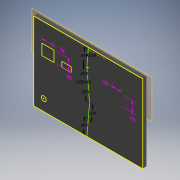
# Autodesk Inventor part: compnent box front
Saved by Autodesk Inventor 2021 (Build 250183000, 183)
## iProperties
Created: 2023-01-12
Part Number: compnent box front
Material: Generic
Document SubType Name: Modeling
Designer: boyle
Density: 1 g/cm^3
Appearance: Default
Author: boyle
Autodesk Inventor part; units mm, degrees
ref_plane "YZ Plane" through (0, 0, 0) normal (1, 0, 0) x (0, 1, 0)
ref_plane "XZ Plane" through (0, 0, 0) normal (0, 1, 0) x (-1, 0, 0)
ref_plane "XY Plane" through (0, 0, 0) normal (0, 0, 1) x (1, 0, 0)
ref_plane "Work Plane1" through (0, 0, 0) normal (0, 0, 1) x (1, 0, 0)
ref_plane "Work Plane2" through (-88.9, -98.425, 0) normal (0, 0, 1) x (1, 0, 0)
sketch "Sketch1" plane through (0, 0, 0) normal (0, 0, 1) x (1, 0, 0)
  line L0 (19.05, -98.425) -> (-88.9, -98.425) projected
  line L1 (-88.9, -98.425) -> (-88.9, -28.575) projected
  line L2 (-88.9, -28.575) -> (-88.9, 28.575) projected
  line L3 (-88.9, 28.575) -> (-85.09, 28.575) projected
  line L4 (88.9, 28.575) -> (88.9, -28.575) projected
  line L5 (85.09, 28.575) -> (88.9, 28.575) projected
  line L6 (19.05, -28.575) -> (19.05, -98.425) projected
  line L7 (-88.9, 28.575) -> (19.05, 28.575)
  line L8 (19.05, 28.575) -> (19.05, -98.425)
  line L9 (19.05, -98.425) -> (-88.9, -98.425)
  line L10 (-88.9, -98.425) -> (-88.9, 28.575)
  line L11 (15.24, -94.615) -> (-85.09, -94.615) projected
  line L12 (15.24, -94.615) -> (15.24, -28.575) projected
  line L13 (-85.09, -28.575) -> (15.24, -28.575) projected
  line L14 (-85.09, -94.615) -> (-85.09, -28.575) projected
  line L15 (19.05, -28.575) -> (19.05, -98.425) projected
  line L16 (15.24, -28.575) -> (19.05, -28.575) projected
  line L17 (-88.9, -98.425) -> (-88.9, -28.575) projected
  line L18 (19.05, -98.425) -> (-88.9, -98.425) projected
  line L19 (-88.9, 28.575) -> (88.9, 28.575) projected
  line L20 (-88.9, -28.575) -> (19.05, -28.575)
  line L21 (19.05, -28.575) -> (19.05, -98.425)
  line L22 (19.05, -98.425) -> (-88.9, -98.425)
  line L23 (-88.9, -98.425) -> (-88.9, -28.575)
  line L24 (88.9, 28.575) -> (88.9, -98.425)
  line L25 (88.9, -98.425) -> (19.05, -98.425)
  point P0 (0, 0)
  constraints: 20 end point, 4 parallel, 3 perpendicular, 2 horizontal, 1 vertical, 1 other
extrude "Extrusion1" add sketch "Sketch1" along normal blind 6.35 from surface at 0
sketch "Sketch2" plane through (0, 0, 6.35) normal (0, 0, 1) x (1, 0, 0)
  line L0 (-88.9, -98.425) -> (88.9, -98.425) projected
  line L1 (-88.9, -98.425) -> (-88.9, -28.575)
  line L2 (-88.9, 28.575) -> (-88.9, -98.425) projected
  line L3 (88.9, -98.425) -> (88.9, 28.575) projected
  circle A0 centre (-72.4784, -80.0377) radius 3.937
  line L4 (-88.9, 28.575) -> (88.9, 28.575)
  line L5 (88.9, 28.575) -> (88.9, -28.575)
  line L6 (-88.9, -28.575) -> (-88.9, 28.575)
  line L7 (88.9, 28.575) -> (-88.9, 28.575) projected
  line L8 (-43.0622, -12.632) -> (-27.8222, -12.632)
  line L9 (-27.8222, -12.632) -> (-27.8222, -20.76)
  line L10 (-27.8222, -20.76) -> (-43.0622, -20.76)
  line L11 (-43.0622, -20.76) -> (-43.0622, -12.632)
  line L12 (-43.0622, -12.632) -> (-27.8222, -20.76) construction
  line L13 (-27.8222, -12.632) -> (-43.0622, -20.76) construction
  line L14 (-75.5122, -3.16) -> (-55.7622, -3.16)
  line L15 (-55.7622, -3.16) -> (-55.7622, -20.76)
  line L16 (-55.7622, -20.76) -> (-75.5122, -20.76)
  line L17 (-75.5122, -20.76) -> (-75.5122, -3.16)
  line L18 (-75.5122, -3.16) -> (-55.7622, -20.76) construction
  line L19 (-55.7622, -3.16) -> (-75.5122, -20.76) construction
  line L20 (-62.5275, -46.3991) -> (-26.5275, -46.3991)
  line L21 (-26.5275, -46.3991) -> (-26.5275, -82.3991)
  line L22 (-26.5275, -82.3991) -> (-62.5275, -82.3991)
  line L23 (-62.5275, -46.3991) -> (-26.5275, -82.3991) construction
  line L24 (-26.5275, -46.3991) -> (-62.5275, -82.3991) construction
  line L25 (-62.5275, -46.3991) -> (-62.5275, -82.3991)
  line L26 (-44.5275, -46.3991) -> (-44.5275, -49.3991)
  line L27 (-44.5275, -49.3991) -> (-62.5275, -49.3991)
  line L28 (-44.5275, -49.3991) -> (-26.5275, -49.3991)
  line L29 (-44.5275, -49.3991) -> (-44.5275, -52.3991)
  line L30 (-44.5275, -52.3991) -> (-62.5275, -52.3991)
  line L31 (-44.5275, -52.3991) -> (-26.5275, -52.3991)
  line L32 (-44.5275, -52.3991) -> (-44.5275, -55.3991)
  line L33 (-44.5275, -55.3991) -> (-62.5275, -55.3991)
  line L34 (-44.5275, -55.3991) -> (-26.5275, -55.3991)
  line L35 (-44.5275, -55.3991) -> (-44.5275, -58.3991)
  line L36 (-44.5275, -58.3991) -> (-62.5275, -58.3991)
  line L37 (-44.5275, -58.3991) -> (-26.5275, -58.3991)
  line L38 (-44.5275, -58.3991) -> (-44.5275, -61.3991)
  line L39 (-44.5275, -61.3991) -> (-62.5275, -61.3991)
  line L40 (-44.5275, -61.3991) -> (-26.5275, -61.3991)
  line L41 (-44.5275, -61.3991) -> (-44.5275, -64.3991)
  line L42 (-44.5275, -64.3991) -> (-62.5275, -64.3991)
  line L43 (-44.5275, -64.3991) -> (-26.5275, -64.3991)
  line L44 (-44.5275, -64.3991) -> (-44.5275, -67.3991)
  line L45 (-44.5275, -67.3991) -> (-62.5275, -67.3991)
  line L46 (-44.5275, -67.3991) -> (-26.5275, -67.3991)
  line L47 (-44.5275, -67.3991) -> (-44.5275, -70.3991)
  line L48 (-44.5275, -70.3991) -> (-62.5275, -70.3991)
  line L49 (-44.5275, -70.3991) -> (-26.5275, -70.3991)
  line L50 (-44.5275, -70.3991) -> (-44.5275, -73.3991)
  line L51 (-44.5275, -73.3991) -> (-62.5275, -73.3991)
  line L52 (-44.5275, -73.3991) -> (-26.5275, -73.3991)
  line L53 (-44.5275, -73.3991) -> (-44.5275, -76.3991)
  line L54 (-44.5275, -76.3991) -> (-62.5275, -76.3991)
  line L55 (-44.5275, -76.3991) -> (-26.5275, -76.3991)
  line L56 (-44.5275, -76.3991) -> (-44.5275, -79.3991)
  line L57 (-44.5275, -79.3991) -> (-62.5275, -79.3991)
  line L58 (-44.5275, -79.3991) -> (-26.5275, -79.3991)
  line L59 (-44.5275, -79.3991) -> (-44.5275, -82.3991)
  line L60 (-44.5275, -82.3991) -> (-62.5275, -82.3991)
  line L61 (-44.5275, -82.3991) -> (-26.5275, -82.3991)
  line L62 (-43.0622, -20.76) -> (-55.7622, -20.76)
  point P0 (-65.6372, -11.96)
  point P1 (-62.5275, -67.3991)
  point P2 (-26.5275, -70.3991)
  point P3 (-26.5275, -67.3991)
  point P4 (-26.5275, -76.3991)
  point P5 (-26.5275, -73.3991)
  point P6 (-26.5275, -79.3991)
  point P7 (-26.5275, -61.3991)
  point P8 (-26.5275, -58.3991)
  point P9 (-26.5275, -55.3991)
  point P10 (-26.5275, -52.3991)
  dimension "d2" = 69.85
  dimension "d5" = 7.874
  dimension "d8" = 15.24
  dimension "d9" = 8.128
  dimension "d12" = 19.75
  dimension "d13" = 17.6
  dimension "d34" = 36
  dimension "d35" = 36
  dimension "d39" = 3
  dimension "d40" = 3
  dimension "d41" = 3
  dimension "d42" = 3
  dimension "d43" = 3
  dimension "d44" = 3
  dimension "d45" = 3
  dimension "d46" = 3
  dimension "d47" = 3
  dimension "d48" = 3
  dimension "d49" = 3
  dimension "d50" = 3
  dimension "d68" = 12.7
  constraints: 118 end point, 13 vertical, 6 parallel, 6 perpendicular, 5 horizontal, 4 point on line, 3 midpoint, 1 centre point
  measures "d2" distance of L0.start L1.end
  measures "d5" diameter of A0
  measures "d8" distance of L8.start L8.end
  measures "d9" distance of L8.end L9.end
  measures "d12" distance of L14.start L14.end
  measures "d13" distance of L14.end L15.end
  measures "d34" distance of L21.end L22.end
  measures "d35" distance of L20.end L21.end
  measures "d39" distance of L26.start L26.end
  measures "d40" distance of L29.start L29.end
  measures "d41" distance of L32.start L32.end
  measures "d42" distance of L35.start L35.end
  measures "d43" distance of L38.start L38.end
  measures "d44" distance of L41.start L41.end
  measures "d45" distance of L44.start L44.end
  measures "d46" distance of L47.start L47.end
  measures "d47" distance of L50.start L50.end
  measures "d48" distance of L53.start L53.end
  measures "d49" distance of L56.start L56.end
  measures "d50" distance of L59.start L59.end
  measures "d68" distance of L10.end L62.end
extrude "Extrusion2" [suppressed]
sketch "Sketch3" plane through (0, 0, 6.35) normal (0, 0, 1) x (1, 0, 0)
  line L0 (88.9, 28.575) -> (-88.9, 28.575) projected
  line L1 (-88.9, -98.425) -> (88.9, -98.425) projected
  line L2 (-88.9, -98.425) -> (88.9, -98.425) projected
  line L3 (0, 25.29) -> (30.48, 25.29) construction
  line L4 (0, 25.29) -> (-2.1566, 0.6394)
  line L5 (0, 25.29) -> (24.7447, 25.29) construction
  line L6 (-2.1566, 0.6394) -> (0, -24.0111)
  line L7 (0, -24.0111) -> (2.1566, -48.6616)
  line L8 (2.1566, -48.6616) -> (0, -73.3121)
  line L9 (0, -73.3121) -> (-2.1566, -97.9626)
  line L10 (0, 25.29) -> (0, 28.575)
  line L11 (-2.1566, -97.9626) -> (-2.1566, -98.425)
  line L12 (-88.9, 28.575) -> (-88.9, -98.425) projected
  line L13 (-27.8222, -20.76) -> (-43.0622, -20.76) projected
  line L14 (-43.0622, -20.76) -> (-43.0622, -12.632) projected
  line L15 (-43.0622, -12.632) -> (-27.8222, -12.632) projected
  line L16 (-27.8222, -12.632) -> (-27.8222, -20.76) projected
  line L17 (-55.7622, -3.16) -> (-55.7622, -20.76) projected
  line L18 (-55.7622, -20.76) -> (-75.5122, -20.76) projected
  line L19 (-75.5122, -20.76) -> (-75.5122, -3.16) projected
  line L20 (-75.5122, -3.16) -> (-55.7622, -3.16) projected
  circle A0 centre (-72.4784, -80.0377) radius 3.937 projected
  line L21 (88.9, 28.575) -> (-88.9, 28.575) projected
  line L22 (-88.9, 28.575) -> (-88.9, -98.425) projected
  line L23 (-88.9, -98.425) -> (88.9, -98.425) projected
  line L24 (88.9, -98.425) -> (88.9, 28.575) projected
  point P0 (0, 0)
  dimension "d21" = 24.7447
  dimension "d22" = 95
  dimension "d23" = 24.7447
  dimension "d24" = 24.7447
  dimension "d25" = 180
  dimension "d26" = 24.7447
  dimension "d27" = 24.7447
  constraints: 18 end point, 2 horizontal, 2 point on line, 1 collinear, 1 equal length, 1 midpoint, 1 perpendicular
  measures "d21" distance of L3.start L4.end
  measures "d22" angle of L4 L5
  measures "d23" distance of L4.end L6.end
  measures "d24" distance of L6.end L7.end
  measures "d25" angle of L7 L6
  measures "d26" distance of L7.end L8.end
  measures "d27" distance of L8.end L9.end
body "Solid1"
